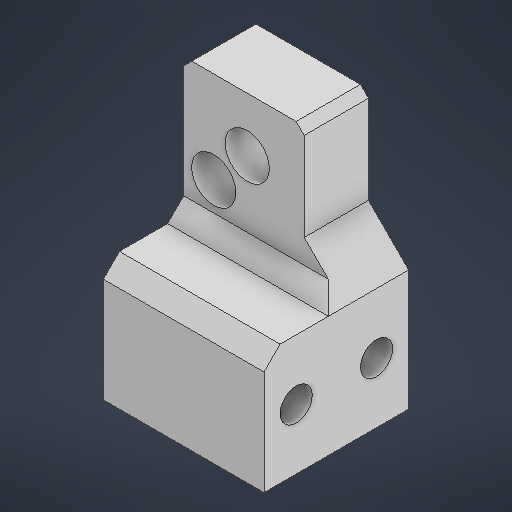
# Autodesk Inventor part: 滚纸
Saved by Autodesk Inventor 2025 (Build 290162000, 162)
## iProperties
Created: 2026-04-27
Part Number: 滚纸
Material: 常规
Document SubType Name: Modeling
Designer: XH
Density: 1 g/cm^3
Appearance: 默认
Author: XH
Autodesk Inventor part; units mm, degrees
ref_plane "YZ Plane" through (0, 0, 0) normal (1, 0, 0) x (0, 1, 0)
ref_plane "XZ Plane" through (0, 0, 0) normal (0, 1, 0) x (-1, 0, 0)
ref_plane "XY Plane" through (0, 0, 0) normal (0, 0, 1) x (1, 0, 0)
sketch "草图1" plane through (0, 0, 0) normal (0, 0, 1) x (1, 0, 0)
  circle A0 centre (0.6467, -2.2689) radius 2.75
  circle A1 centre (4.8161, 2.4002) radius 2.5 construction
  circle A2 centre (4.8161, 2.4002) radius 2.5 construction
  circle A3 centre (4.8161, 2.4002) radius 2.5 construction
  line L0 (16.9048, -7.8392) -> (-3.0952, -7.8392)
  line L1 (-3.0952, -7.8392) -> (-3.0952, -22.8392)
  line L2 (-3.0952, -22.8392) -> (16.9048, -22.8392)
  line L3 (16.9048, -22.8392) -> (16.9048, -7.8392)
  line L4 (16.9048, -6.8375) -> (16.9048, -82.9867) projected
  line L5 (-1.0952, -7.8392) -> (16.9048, -7.8392) projected
  line L6 (-3.0952, 9.1608) -> (11.9048, 9.1608)
  line L7 (11.9048, 9.1608) -> (11.9048, -22.8392)
  line L8 (11.9048, -22.8392) -> (-3.0952, -22.8392)
  line L9 (-3.0952, -22.8392) -> (-3.0952, 9.1608)
  circle A4 centre (4.8161, 2.4002) radius 2.75
  point P0 (-3.0952, -7.8392)
  point P1 (11.9048, -7.8392)
  dimension "d2" = 15
  dimension "d3" = 20
  dimension "d4" = 15
  dimension "d5" = 17
  dimension "d26" = 5.5
  dimension "d28" = 5.5
  constraints: 16 end point, 4 parallel, 3 centre point, 2 coincident, 2 collinear, 2 horizontal, 2 perpendicular, 1 concentric, 1 point on line
  measures "d2" distance between parallel lines of L2 L0
  measures "d3" distance between parallel lines of L3 L1
  measures "d4" distance of L6.start L6.end
  measures "d5" distance between parallel lines of L0 L6
  measures "d26" diameter of A0
  measures "d28" diameter of A4
extrude "拉伸1" add sketch "草图1" against normal blind 12
move faces "移动1" translate (0, 0, -4) faces at (8.5714, -17.8392, 0)
sketch "草图3" plane through (-3.0952, -22.8392, -4) normal (0, 0, 1) x (1, 0, 0)
  line L0 (20, 15) -> (20, 0) projected
  line L1 (0, 0) -> (0, 32) projected
  line L2 (20, 0) -> (0, 0)
  line L3 (0, 0) -> (0, 15)
  line L4 (0, 15) -> (20, 15)
  line L5 (20, 15) -> (20, 0)
  line L6 (20, 15) -> (15, 15) projected
  point P0 (3.0952, 22.8392)
  constraints: 8 end point, 2 parallel, 1 collinear, 1 horizontal, 1 perpendicular, 1 point on line
extrude "拉伸2" add sketch "草图3" along normal blind 10
chamfer "倒角1" distance 5 angle 45 1 edges at (11.9048, -7.8392, -8)
chamfer "倒角2" distance 1 angle 45 2 edges at (-3.0952, 9.1608, -8) (11.9048, 9.1608, -8)
sketch "草图4" plane through (16.9048, -22.8392, 6) normal (1, 0, 0) x (0, 0, -1)
  circle A0 centre (4, 7.5) radius 2
  line L0 (0, 15) -> (0, 0) projected
  line L1 (0, 7.5) -> (18, 7.5)
  line L2 (18, 0) -> (18, 31) projected
  circle A1 centre (14, 7.5) radius 2
  line L3 (0, 0) -> (0, 15) projected
  point P0 (6, 22.8392)
  point P1 (0, 7.5)
  dimension "d17" = 4
  dimension "d18" = 4
  dimension "d19" = 10
  dimension "d20" = 4
  constraints: 3 point on line, 2 centre point, 2 end point, 2 midpoint, 1 horizontal
  measures "d17" diameter of A0
  measures "d18" diameter of A1
  measures "d19" distance of A1.centre A0.centre
  measures "d20" distance of A0.centre point (0, 7.5)
extrude "拉伸3" cut sketch "草图4" against normal blind 5
chamfer "倒角3" distance 2 angle 45 2 edges at (6.9048, -7.8392, 6) (6.9047, -7.8392, -4)
